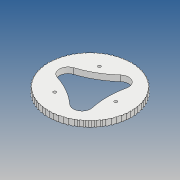
# Autodesk Inventor part: Plato Correa 2
Saved by Autodesk Inventor 2017 (Build 210142000, 142)
## iProperties
Part Number: Plato Correa 2
Material: Genérico
Document SubType Name: Modeling
Designer: FABLAB
Density: 1 g/cm^3
Appearance: Blanco
Author: FABLAB
Autodesk Inventor part; units mm, degrees
ref_plane "YZ Plane" through (0, 0, 0) normal (1, 0, 0) x (0, 1, 0)
ref_plane "XZ Plane" through (0, 0, 0) normal (0, 1, 0) x (-1, 0, 0)
ref_plane "XY Plane" through (0, 0, 0) normal (0, 0, 1) x (1, 0, 0)
sketch "Boceto1" plane through (0, 0, 0) normal (0, 0, 1) x (1, 0, 0)
  circle A0 centre (26.75, 0) radius 1.5 projected
  arc A1 (20.168, 17.783) -> (20.168, -17.783) centre (101.6471, 0) ccw projected
  arc A2 (5.3165, -26.3575) -> (20.168, -17.783) centre (11.375, -19.7021) ccw projected
  arc A3 (5.3165, -26.3575) -> (-25.4845, -8.5745) centre (-50.8235, -88.0289) ccw projected
  arc A4 (-25.4845, 8.5745) -> (-25.4845, -8.5745) centre (-22.75, 0) ccw projected
  arc A5 (-25.4845, 8.5745) -> (5.3165, 26.3575) centre (-50.8235, 88.0289) ccw projected
  arc A6 (20.168, 17.783) -> (5.3165, 26.3575) centre (11.375, 19.7021) ccw projected
  arc A7 (43.9264, -13.8119) -> (-43.9264, -13.8119) centre (0, 0) ccw construction
  circle A8 centre (-13.375, 23.1662) radius 1.5 projected
  circle A9 centre (-13.375, -23.1662) radius 1.5 projected
  circle A10 centre (42.7967, 0) radius 0.75
  line L0 (0, 0) -> (0, -72) construction
  arc A11 (-23.3242, -79.3339) -> (23.3242, -79.3339) centre (0, -72) ccw construction
  line L1 (23.3242, -79.3339) -> (43.9264, -13.8119) construction
  line L2 (-23.3242, -79.3339) -> (-43.9264, -13.8119) construction
  circle A12 centre (42.5907, 4.1948) radius 0.75
  circle A13 centre (41.9744, 8.3492) radius 0.75
  circle A14 centre (40.9539, 12.4232) radius 0.75
  circle A15 centre (39.539, 16.3776) radius 0.75
  circle A16 centre (37.7433, 20.1742) radius 0.75
  circle A17 centre (35.5842, 23.7766) radius 0.75
  circle A18 centre (33.0823, 27.15) radius 0.75
  circle A19 centre (30.2619, 30.2619) radius 0.75
  circle A20 centre (27.15, 33.0823) radius 0.75
  circle A21 centre (23.7766, 35.5842) radius 0.75
  circle A22 centre (20.1742, 37.7433) radius 0.75
  circle A23 centre (16.3776, 39.539) radius 0.75
  circle A24 centre (12.4232, 40.9539) radius 0.75
  circle A25 centre (8.3492, 41.9744) radius 0.75
  circle A26 centre (4.1948, 42.5907) radius 0.75
  circle A27 centre (0, 42.7967) radius 0.75
  circle A28 centre (-4.1948, 42.5907) radius 0.75
  circle A29 centre (-8.3492, 41.9744) radius 0.75
  circle A30 centre (-12.4232, 40.9539) radius 0.75
  circle A31 centre (-16.3776, 39.539) radius 0.75
  circle A32 centre (-20.1742, 37.7433) radius 0.75
  circle A33 centre (-23.7766, 35.5842) radius 0.75
  circle A34 centre (-27.15, 33.0823) radius 0.75
  circle A35 centre (-30.2619, 30.2619) radius 0.75
  circle A36 centre (-33.0823, 27.15) radius 0.75
  circle A37 centre (-35.5842, 23.7766) radius 0.75
  circle A38 centre (-37.7433, 20.1742) radius 0.75
  circle A39 centre (-39.539, 16.3776) radius 0.75
  circle A40 centre (-40.9539, 12.4232) radius 0.75
  circle A41 centre (-41.9744, 8.3492) radius 0.75
  circle A42 centre (-42.5907, 4.1948) radius 0.75
  circle A43 centre (-42.7967, 0) radius 0.75
  circle A44 centre (-42.5907, -4.1948) radius 0.75
  circle A45 centre (-41.9744, -8.3492) radius 0.75
  circle A46 centre (-40.9539, -12.4232) radius 0.75
  circle A47 centre (-39.539, -16.3776) radius 0.75
  circle A48 centre (-37.7433, -20.1742) radius 0.75
  circle A49 centre (-35.5842, -23.7766) radius 0.75
  circle A50 centre (-33.0823, -27.15) radius 0.75
  circle A51 centre (-30.2619, -30.2619) radius 0.75
  circle A52 centre (-27.15, -33.0823) radius 0.75
  circle A53 centre (-23.7766, -35.5842) radius 0.75
  circle A54 centre (-20.1742, -37.7433) radius 0.75
  circle A55 centre (-16.3776, -39.539) radius 0.75
  circle A56 centre (-12.4232, -40.9539) radius 0.75
  circle A57 centre (-8.3492, -41.9744) radius 0.75
  circle A58 centre (-4.1948, -42.5907) radius 0.75
  circle A59 centre (0, -42.7967) radius 0.75
  circle A60 centre (4.1948, -42.5907) radius 0.75
  circle A61 centre (8.3492, -41.9744) radius 0.75
  circle A62 centre (12.4232, -40.9539) radius 0.75
  circle A63 centre (16.3776, -39.539) radius 0.75
  circle A64 centre (20.1742, -37.7433) radius 0.75
  circle A65 centre (23.7766, -35.5842) radius 0.75
  circle A66 centre (27.15, -33.0823) radius 0.75
  circle A67 centre (30.2619, -30.2619) radius 0.75
  circle A68 centre (33.0823, -27.15) radius 0.75
  circle A69 centre (35.5842, -23.7766) radius 0.75
  circle A70 centre (37.7433, -20.1742) radius 0.75
  circle A71 centre (39.539, -16.3776) radius 0.75
  circle A72 centre (40.9539, -12.4232) radius 0.75
  circle A73 centre (41.9744, -8.3492) radius 0.75
  arc A74 (-43.9264, -13.8119) -> (43.9264, -13.8119) centre (0, 0) ccw construction
  circle A75 centre (42.5907, -4.1948) radius 0.75
  circle A76 centre (0, 0) radius 42.7967
  circle A77 centre (0, 0) radius 42.0467 construction
  dimension "d0" = 92.0935
  dimension "d9" = 1.5
  dimension "d11" = 72
  dimension "d20" = 61.9148
  dimension "d21" = 172.7159
  dimension "d22" = 68.6847
  dimension "d23" = 24.45
  dimension "d26" = 360
  dimension "d28" = 4.1999
  dimension "d31" = 4
  constraints: 68 centre point, 7 tangent, 6 end point, 6 point on circle, 4 coincident, 2 horizontal alignment, 1 vertical, 131 other
  measures "d0" diameter of A7
  measures "d9" diameter of A10
  measures "d11" distance of L0.start L0.end
  measures "d22" distance of L1.start L1.end
  measures "d23" radius of A11
  measures "d28" distance of A18.centre A19.centre
  measures "d31" radial gap between concentric circles of A77 A7
extrude "Extrusión1" add sketch "Boceto1" along normal blind 6
sketch "Boceto2" plane through (0, 0, 6) normal (0, 0, 1) x (1, 0, 0)
  circle A0 centre (0, 0) radius 41.5
  arc A1 (20.168, 17.783) -> (20.168, -17.783) centre (101.6471, 0) ccw
  arc A2 (20.168, 17.783) -> (5.3165, 26.3575) centre (11.375, 19.7021) ccw projected
  arc A3 (-25.4845, 8.5745) -> (5.3165, 26.3575) centre (-50.8235, 88.0289) ccw
  arc A4 (-25.4845, 8.5745) -> (-25.4845, -8.5745) centre (-22.75, 0) ccw
  arc A5 (5.3165, -26.3575) -> (-25.4845, -8.5745) centre (-50.8235, -88.0289) ccw projected
  arc A6 (5.3165, -26.3575) -> (20.168, -17.783) centre (11.375, -19.7021) ccw projected
  circle A7 centre (-13.375, -23.1662) radius 1.5 projected
  circle A8 centre (-13.375, 23.1662) radius 1.5 projected
  circle A9 centre (26.75, 0) radius 1.5 projected
  dimension "d30" = 83
  constraints: 6 point on circle, 4 centre point, 1 coincident, 11 other
  measures "d30" diameter of A0
sketch "Boceto3" plane through (0, 0, 0) normal (0, 0, -1) x (-1, 0, 0)
  circle A0 centre (0, 0) radius 41.5 projected
  circle A1 centre (0, 0) radius 36
  point P0 (0, 0)
  dimension "d6" = 5.5
  constraints: 1 centre point
  measures "d6" radial gap between concentric circles of A0 A1
